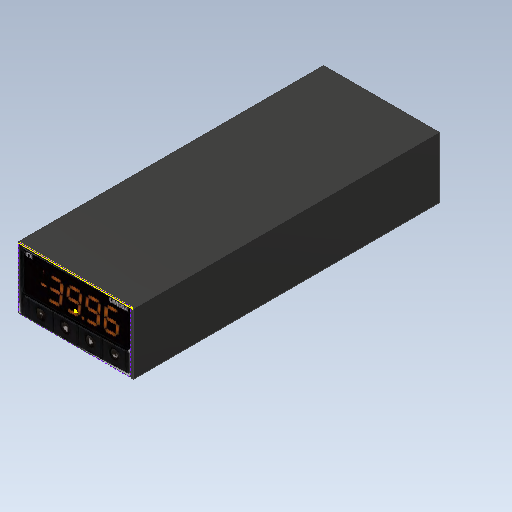
# Autodesk Inventor part: Omega_CN32PT-330
Saved by Autodesk Inventor 2020 (Build 240168000, 168)
## iProperties
Created: 2018-08-16
Part Number: Omega_CN32PT-330
Material: ABS Plastic
Document SubType Name: Modeling
Designer: Rich
Density: 1.06 g/cm^3
Appearance: Smooth - Black
Author: Rich
Autodesk Inventor part; units mm, degrees
ref_plane "YZ Plane" through (0, 0, 0) normal (1, 0, 0) x (0, 1, 0)
ref_plane "XZ Plane" through (0, 0, 0) normal (0, 1, 0) x (-1, 0, 0)
ref_plane "XY Plane" through (0, 0, 0) normal (0, 0, 1) x (1, 0, 0)
sketch "Sketch1" plane through (0, 0, 0) normal (0, 0, 1) x (1, 0, 0)
  line L0 (-24, 12.7) -> (24, 12.7)
  line L1 (24, 12.7) -> (24, -12.7)
  line L2 (24, -12.7) -> (-24, -12.7)
  line L3 (-24, -12.7) -> (-24, 12.7)
  line L4 (-24, 12.7) -> (24, -12.7) construction
  line L5 (24, 12.7) -> (-24, -12.7) construction
  point P0 (0, 0)
  dimension "d0" = 48
  dimension "d1" = 25.4
  constraints: 12 end point, 2 midpoint, 2 parallel, 1 horizontal, 1 perpendicular
  measures "d0" distance of L1.end L2.end
  measures "d1" distance of L0.end L1.end
extrude "Extrusion1" add sketch "Sketch1" against normal blind 127
sketch "Sketch2" plane through (0, 0, 0) normal (0, 0, 1) x (1, 0, 0)
  line L0 (-24, 12.7) -> (24, 12.7) projected
  line L1 (-24, 12.7) -> (22.7997, 12.7665) construction
  line L2 (22.7997, 12.7665) -> (22.836, -12.7908) construction
  line L3 (22.836, -12.7908) -> (-23.9637, -12.8573) construction
  line L4 (-23.9637, -12.8573) -> (-24, 12.7) construction
  point P0 (0, 0)
  constraints: 2 other
body "Solid1"
